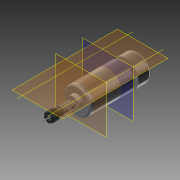
# Autodesk Inventor part: vreteno
Saved by Autodesk Inventor 2013 (Build 170138000, 138)
## iProperties
Created: 2014-01-21
Part Number: vreteno
Material: Všeobecné
Document SubType Name: Modeling
Designer: martin
Density: 1 g/cm^3
Author: martin
Autodesk Inventor part; units mm, degrees
ref_plane "YZ Plane" through (0, 0, 0) normal (1, 0, 0) x (0, 1, 0)
ref_plane "XZ Plane" through (0, 0, 0) normal (0, 1, 0) x (-1, 0, 0)
ref_plane "XY Plane" through (0, 0, 0) normal (0, 0, 1) x (1, 0, 0)
sketch "Náčrt2" plane through (0, 0, 0) normal (0, 1, 0) x (-1, 0, 0)
  circle A0 centre (0, 0) radius 26
  dimension "d1" = 26
  constraints: 1 centre point, 1 coincident
  measures "d1" radius of A0
extrude "Vysunutí1" add sketch "Náčrt2" along normal blind 90
sketch "Náčrt3" plane through (0, 0, 0) normal (0, -1, 0) x (1, 0, 0)
  circle A0 centre (0, 0) radius 26 projected
  circle A1 centre (0, 0) radius 13
  dimension "d4" = 13
  constraints: 1 centre point, 1 coincident
  measures "d4" radius of A1
extrude "Vysunutí2" add sketch "Náčrt3" along normal blind 7 contours A1
fillet "Zaoblení1" radius 3 1 edges at (26, 0, 0)
fillet "Zaoblení2" radius 3 1 edges at (26, 90, 0)
sketch "Náčrt4" plane through (0, -7, 0) normal (0, -1, 0) x (1, 0, 0)
  circle A0 centre (0, 0) radius 13 projected
  circle A1 centre (0, 0) radius 4
  dimension "d9" = 4
  constraints: 1 centre point, 1 coincident
  measures "d9" radius of A1
extrude "Vysunutí3" add sketch "Náčrt4" along normal blind 5 contours A1
chamfer "Zkosení1" distance 7 angle 10 1 edges at (-13, -7, 0) measured on face at (-13, -6.5, 0)
sketch "Náčrt5" plane through (0, -12, 0) normal (0, -1, 0) x (1, 0, 0)
  circle A0 centre (0, 0) radius 4 construction
  circle A1 centre (0, 0) radius 8
  dimension "d15" = 8
  constraints: 1 centre point, 1 coincident
  measures "d15" radius of A1
extrude "Vysunutí4" add sketch "Náčrt5" along normal blind 44
sketch "Náčrt6" plane through (0, -56, 0) normal (0, -1, 0) x (1, 0, 0)
  circle A0 centre (0, 0) radius 8 projected
  circle A1 centre (0, 0) radius 9.5
  dimension "d19" = 9.5
  constraints: 1 centre point, 1 coincident
  measures "d19" radius of A1
extrude "Vysunutí5" add sketch "Náčrt6" against normal blind 13
sketch "Náčrt7" plane through (0, -56, 0) normal (0, -1, 0) x (1, 0, 0)
  circle A0 centre (0, 0) radius 9.5 projected
  circle A1 centre (0, 0) radius 5
  dimension "d22" = 5
  constraints: 1 centre point, 1 coincident
  measures "d22" radius of A1
extrude "Vysunutí6" cut sketch "Náčrt7" against normal blind 3 contours A1
sketch "Náčrt8" plane through (0, -56, 0) normal (0, -1, 0) x (1, 0, 0)
  circle A0 centre (0, 0) radius 9.5 projected
  line L0 (0, 9.5) -> (8.2272, 4.75)
  line L1 (8.2272, 4.75) -> (8.2272, -4.75)
  line L2 (8.2272, -4.75) -> (0, -9.5)
  line L3 (0, -9.5) -> (-8.2272, -4.75)
  line L4 (-8.2272, -4.75) -> (-8.2272, 4.75)
  line L5 (-8.2272, 4.75) -> (0, 9.5)
  constraints: 12 end point, 1 coincident, 1 vertical alignment, 14 other
extrude "Vysunutí7" cut sketch "Náčrt8" against normal blind 5 contours A0 L1 | L0 A0 | A0 L2 | L5 A0 | A0 L3 | L4 A0
sketch "Náčrt9" plane through (0, -53, 0) normal (0, -1, 0) x (1, 0, 0)
  circle A0 centre (0, 0) radius 5 projected
  circle A1 centre (0, 0) radius 1.5875
  dimension "d27" = 3.175
  constraints: 1 centre point, 1 coincident
  measures "d27" diameter of A1
extrude "Vysunutí8" add sketch "Náčrt9" along normal blind 5 contours A1
sketch "Náčrt10" plane through (0, -58, 0) normal (0, -1, 0) x (1, 0, 0)
  circle A0 centre (0, 0) radius 1.5875 projected
  circle A1 centre (0, 0) radius 1
  dimension "d30" = 2
  constraints: 1 centre point, 1 coincident
  measures "d30" diameter of A1
extrude "Vysunutí9" add sketch "Náčrt10" along normal blind 10 contours A1
chamfer "Zkosení2" distance 0.52 distance2 3 1 edges at (-1.5875, -58, 0) measured on face at (-1.4875, -58, 0)
ref_plane "Pracovní rovina1" through (4, -12, -6.9282) normal (0.5, 0, -0.8660254) x (0, 1, 0)
sketch "Náčrt11" plane through (4, -12, -6.9282) normal (0.5, 0, -0.8660254) x (0, 1, 0)
  line L0 (-12.65, -6.5) -> (-6.65, -6.5)
  line L1 (-6.65, -6.5) -> (-6.65, 6.5) construction
  line L2 (-6.65, 6.5) -> (-12.65, 6.5)
  line L3 (-12.65, 6.5) -> (-12.65, -6.5) construction
  line L4 (-12.65, -6.5) -> (-6.65, 6.5) construction
  line L5 (-6.65, -6.5) -> (-12.65, 6.5) construction
  line L6 (-12.65, 6.5) -> (-6.65, 6.5)
  line L7 (-6.65, 6.5) -> (-6.65, 8.9956)
  line L8 (-6.65, 8.9956) -> (-12.65, 8.9956)
  line L9 (-12.65, 8.9956) -> (-12.65, 6.5)
  line L10 (-12.65, -6.5) -> (-6.65, -6.5)
  line L11 (-6.65, -6.5) -> (-6.65, -9.8192)
  line L12 (-6.65, -9.8192) -> (-12.65, -9.8192)
  line L13 (-12.65, -9.8192) -> (-12.65, -6.5)
  point P0 (12, 0)
  point P1 (-9.65, 0)
  dimension "d36" = 6
  dimension "d37" = 13
  constraints: 28 end point, 6 parallel, 3 horizontal, 3 perpendicular, 2 midpoint
  measures "d36" distance of L2.end L1.end
  measures "d37" distance of L1.end L0.end
extrude "Vysunutí10" cut sketch "Náčrt11" against normal through all
thread "Závit1" size "M16x2" class "6g" standard "ANSI Metric M Profile" length 10
sketch "Náčrt12" plane through (0, 90, 0) normal (0, 1, 0) x (1, 0, 0)
  circle A0 centre (0, 0) radius 23 projected
  circle A1 centre (0, 0) radius 4
  dimension "d42" = 8
  constraints: 1 centre point, 1 coincident
  measures "d42" diameter of A1
extrude "Vysunutí11" add sketch "Náčrt12" along normal blind 30 contours A1
sketch "Náčrt13" plane through (0, 120, 0) normal (0, 1, 0) x (1, 0, 0)
  circle A0 centre (0, 0) radius 4 projected
  circle A1 centre (0, 0) radius 26
  dimension "d45" = 52
  constraints: 1 centre point, 1 coincident
  measures "d45" diameter of A1
extrude "Vysunutí12" add sketch "Náčrt13" against normal blind 25
fillet "Zaoblení3" radius 5 1 edges at (-26, 120, 0)
sketch "Náčrt14" plane through (0, 120, 0) normal (0, 1, 0) x (1, 0, 0)
  circle A0 centre (0, 0) radius 17
  circle A1 centre (0, 0) radius 4 projected
  dimension "d49" = 34
  constraints: 1 centre point, 1 coincident
  measures "d49" diameter of A0
extrude "Vysunutí13" cut sketch "Náčrt14" against normal blind 4
ref_plane "Pracovní rovina2" through (0, 3, 0) normal (0, -1, 0) x (1, 0, 0)
sketch "Náčrt15" plane through (0, 3, 0) normal (0, -1, 0) x (1, 0, 0)
  circle A0 centre (0, 0) radius 26
  circle A1 centre (0, 0) radius 36
  circle A2 centre (0, 0) radius 45 construction
  line L0 (-30, 33.541) -> (30, 33.541) construction
  circle A3 centre (-30, 33.541) radius 5.1
  circle A4 centre (30, 33.541) radius 5.1
  arc A5 (-30, 48.641) -> (-36, 19.6843) centre (-30, 33.541) ccw
  arc A6 (36, 19.6843) -> (30, 48.641) centre (30, 33.541) ccw
  line L1 (-30, 48.641) -> (30, 48.641)
  line L2 (-36, 0) -> (-36, 19.6843)
  line L3 (36, 0) -> (36, 19.6843)
  dimension "d52" = 26
  dimension "d53" = 36
  dimension "d54" = 45
  dimension "d55" = 60
  dimension "d56" = 5.1
  dimension "d57" = 10
  constraints: 9 point on circle, 8 end point, 7 centre point, 6 coincident, 4 tangent, 2 equal radius, 2 parallel, 1 horizontal, 1 perpendicular
  measures "d52" radius of A0
  measures "d53" radius of A1
  measures "d54" radius of A2
  measures "d55" distance of L0.start L0.end
  measures "d56" radius of A3
  measures "d57" radial gap between concentric circles of A5 A3
extrude "Vysunutí14" add sketch "Náčrt15" against normal blind 10 separate body
ref_plane "Pracovní rovina5" through (0, 75, 0) normal (0, 1, 0) x (1, 0, 0)
ref_plane "Pracovní rovina4" through (0, 8, 0) normal (0, -1, 0) x (1, 0, 0)
sketch "Náčrt17" plane through (0, 8, 0) normal (0, -1, 0) x (1, 0, 0)
  circle A0 centre (-30, 33.541) radius 5.1 projected
  circle A1 centre (30, 33.541) radius 5.1 projected
  circle A2 centre (-30, 33.541) radius 7.5
  circle A3 centre (30, 33.541) radius 7.5
  point P0 (0, 0)
  dimension "d62" = 7.5
  constraints: 2 centre point, 2 coincident, 1 equal radius
  measures "d62" radius of A2
extrude "Vysunutí15" add sketch "Náčrt17" against normal blind 48 separate body
ref_plane "Pracovní rovina6" through (-30, 61, 33.541) normal (0, 1, 0) x (1, 0, 0)
sketch "Náčrt18" plane through (-30, 61, 33.541) normal (0, 1, 0) x (1, 0, 0)
  circle A0 centre (30, 33.541) radius 26 projected
  circle A1 centre (60, 0) radius 5.1 projected
  circle A2 centre (0, 0) radius 5.1 projected
  arc A3 (-6, 13.8568) -> (0, -15.1) centre (0, 0) ccw projected
  line L0 (0, -15.1) -> (60, -15.1) projected
  arc A4 (60, -15.1) -> (66, 13.8568) centre (60, 0) ccw projected
  line L1 (66, 13.8568) -> (66, 33.541) projected
  arc A5 (66, 33.541) -> (-6, 33.541) centre (30, 33.541) ccw projected
  line L2 (-6, 33.541) -> (-6, 13.8568) projected
extrude "Vysunutí16" add sketch "Náčrt18" against normal blind 10 separate body
ref_plane "Pracovní rovina7" through (30, 8, 33.541) normal (0, 0, 1) x (0, 1, 0)
